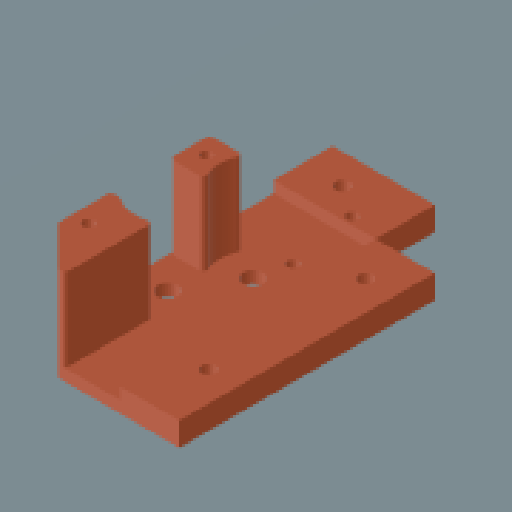
# Autodesk Inventor part: Alpha Idler Assembly
Saved by Autodesk Inventor 2023.2 (Build 272271000, 271)
## iProperties
Created: 2023-02-03
Part Number: Alpha Idler Assembly
Material: ABS Plastic
Document SubType Name: Modeling
Designer: remop
Density: 1.06 g/cm^3
Appearance: Smooth - Light Orange
Author: remop
Autodesk Inventor part; units mm, degrees
ref_plane "YZ Plane" through (0, 0, 0) normal (1, 0, 0) x (0, 1, 0)
ref_plane "XZ Plane" through (0, 0, 0) normal (0, 1, 0) x (-1, 0, 0)
ref_plane "XY Plane" through (0, 0, 0) normal (0, 0, 1) x (1, 0, 0)
sketch "Sketch1" plane through (0, 0, 0) normal (0, 1, 0) x (-1, 0, 0)
  circle A0 centre (25, 36.3) radius 2.5
  circle A1 centre (33, 49.9) radius 2.5
  line L0 (15, 0) -> (15, 15)
  line L1 (15, 15) -> (0, 15)
  line L2 (0, 15) -> (0, 80)
  line L3 (0, 80) -> (41, 80)
  line L4 (41, 80) -> (41, 0)
  line L5 (15, 0) -> (41, 0)
  circle A2 centre (25, 36.3) radius 7.5 construction
  circle A3 centre (33, 49.9) radius 7.5 construction
  point P0 (0, 0)
  dimension "d0" = 5
  dimension "d1" = 15
  dimension "d2" = 25
  dimension "d3" = 21.3
  dimension "d4" = 8
  dimension "d5" = 13.6
  dimension "d12" = 15
  dimension "d46" = 80
  dimension "d47" = 41
  constraints: 12 end point, 6 perpendicular, 4 centre point, 2 coincident, 2 equal radius, 1 horizontal alignment, 1 vertical, 1 vertical alignment
  measures "d0" diameter of A1
  measures "d1" distance of L0.end L1.end
  measures "d2" distance from line of L2 A0.centre
  measures "d3" distance from line of L1 A0.centre
  measures "d4" horizontal distance of A1.centre A0.centre
  measures "d5" vertical distance of A1.centre A0.centre
  measures "d12" diameter of A3
  measures "d46" distance of L3.end L4.end
  measures "d47" distance of L2.end L3.end
extrude "Extrusion1" add sketch "Sketch1" along normal blind 3
sketch "Sketch2" plane through (0, 3, 0) normal (0, 1, 0) x (1, 0, 0)
  line L0 (-41, 0) -> (-41, -80) projected
  line L1 (-41, -80) -> (0, -80) projected
  line L2 (0, -80) -> (0, -15) projected
  line L3 (0, -15) -> (-15, -15) projected
  line L4 (-15, -15) -> (-15, 0) projected
  line L5 (-15, 0) -> (-41, 0) projected
  circle A0 centre (-33, -49.9) radius 2.5 projected
  circle A1 centre (-25, -36.3) radius 2.5 projected
  line L6 (-15, -15) -> (-15, 0) projected
  line L7 (-15, -15) -> (-15, -80)
  line L8 (-15, -15) -> (-41, -15)
  line L9 (-41, 0) -> (-41, -80) projected
  point P0 (0, 0)
  constraints: 4 end point, 3 point on line, 1 perpendicular
extrude "Extrusion2" add sketch "Sketch2" along normal blind 3 contours L5 L4 L8 L0 | L3 L2 L1 L7
sketch "Sketch3" plane through (0, 3, 0) normal (0, 1, 0) x (1, 0, 0)
  circle A0 centre (-25, -36.3) radius 2.5 projected
  circle A1 centre (-33, -49.9) radius 2.5 projected
  line L0 (-15, -80) -> (-15, -15) projected
  line L1 (-15, -15) -> (-41, -15) projected
  line L2 (-41, -15) -> (-41, -80) projected
  line L3 (-41, -80) -> (-15, -80) projected
  circle A2 centre (-25, -36.3) radius 2.5 projected
  circle A3 centre (-25, -36.3) radius 8.5
  circle A4 centre (-33, -49.9) radius 2.5 projected
  circle A5 centre (-33, -49.9) radius 8.5
  line L4 (-31.8739, -31.3) -> (-41, -31.3)
  line L5 (-41, 0) -> (-41, -80) projected
  line L6 (-33, -41.4) -> (-41, -41.4)
  line L7 (-38.3753, -56.4846) -> (-41, -56.4846)
  line L8 (-29, -57.4) -> (-29, -80)
  line L9 (-41, -80) -> (0, -80) projected
  point P0 (0, 0)
  point P1 (-31.727, -41.4959)
  dimension "d15" = 17
  dimension "d16" = 5
  dimension "d19" = 12
  constraints: 8 end point, 4 perpendicular, 4 point on line, 3 point on circle, 2 coincident, 1 centre point, 1 tangent, 4 other
  measures "d16" distance from line of A0.centre L4
  measures "d19" distance between parallel lines of L2 L8
extrude "Extrusion3" add sketch "Sketch3" along normal blind 21 contours L3 L2 L7 A5 L8 | L4 A3 A5 L6 L2
fillet "Fillet1" radius 1 8 edges at (-31.8739, 13.5, 31.3) (-31.727, 13.5, 41.4959) (-41, 13.5, 41.4) (-41, 13.5, 31.3) (-41, 13.5, 56.4846) (-29, 13.5, 57.4) (-29, 13.5, 80) (-38.3753, 13.5, 56.4846)
chamfer "Chamfer1" distance 10 angle 45 1 edges at (-41, 12, 80)
sketch "Sketch4" plane through (0, 24, 0) normal (0, 1, 0) x (1, 0, 0)
  line L0 (-31, -80) -> (-41, -70) projected
  line L1 (-31, -80) -> (-30, -80) projected
  arc A0 (-30, -80) -> (-29, -79) centre (-30, -79) ccw projected
  line L2 (-29, -79) -> (-29, -58.9139) projected
  arc A1 (-29, -58.9139) -> (-30.3158, -57.965) centre (-30, -58.9139) ccw projected
  arc A2 (-38.1184, -56.6862) -> (-30.3158, -57.965) centre (-33, -49.9) ccw projected
  arc A3 (-38.1184, -56.6862) -> (-38.7205, -56.4846) centre (-38.7205, -57.4846) ccw projected
  line L3 (-38.7205, -56.4846) -> (-40, -56.4846) projected
  arc A4 (-40, -56.4846) -> (-41, -57.4846) centre (-40, -57.4846) ccw projected
  line L4 (-41, -57.4846) -> (-41, -70) projected
  arc A5 (-40, -31.3) -> (-41, -32.3) centre (-40, -32.3) ccw projected
  line L5 (-41, -32.3) -> (-41, -40.4) projected
  arc A6 (-41, -40.4) -> (-40, -41.4) centre (-40, -40.4) ccw projected
  line L6 (-40, -41.4) -> (-33.5697, -41.4) projected
  arc A7 (-33.5697, -41.4) -> (-32.6676, -39.9684) centre (-33.5697, -40.4) ccw projected
  arc A8 (-32.7098, -32.7211) -> (-32.6676, -39.9684) centre (-25, -36.3) ccw projected
  arc A9 (-32.7098, -32.7211) -> (-33.6168, -31.3) centre (-33.6168, -32.3) ccw projected
  line L7 (-33.6168, -31.3) -> (-40, -31.3) projected
  point P0 (0, 0)
  point P1 (-37, -36)
  point P2 (-37, -66)
  dimension "d24" = 4
  dimension "d25" = 36
  dimension "d26" = 30
  constraints: 1 vertical alignment
  measures "d24" distance from line of L5 point (-37, -36)
  measures "d25" vertical distance of point (-37, -36) point (0, 0)
  measures "d26" distance of point (-37, -66) point (-37, -36)
hole "Hole1" at (-37, 24, 36) at (-37, 24, 66) direction (0, -1, 0) diameter 2.8 depth 10 tip angle 118
sketch "Sketch5" plane through (0, 0, 0) normal (0, -1, 0) x (1, 0, 0)
  line L0 (-41, 70) -> (-31, 80) projected
  line L1 (-41, 0) -> (-41, 70) projected
  line L2 (-15, 0) -> (-41, 0) projected
  line L3 (-15, 15) -> (-15, 0) projected
  line L4 (0, 15) -> (-15, 15) projected
  line L5 (0, 80) -> (0, 15) projected
  line L6 (-31, 80) -> (0, 80) projected
  circle A0 centre (-33, 49.9) radius 2.5 projected
  circle A1 centre (-25, 36.3) radius 2.5 projected
  point P0 (0, 0)
  point P1 (-31, 7.5)
  point P2 (-7.5, 25)
  point P3 (-7.5, 65)
  dimension "d34" = 7.5
  dimension "d35" = 7.5
  dimension "d36" = 10
  dimension "d37" = 15
  dimension "d38" = 40
  constraints: 1 vertical alignment
  measures "d34" distance from line of L5 point (-7.5, 25)
  measures "d35" distance from line of L2 point (-31, 7.5)
  measures "d36" distance from line of L1 point (-31, 7.5)
  measures "d37" distance from line of L6 point (-7.5, 65)
  measures "d38" distance of point (-7.5, 25) point (-7.5, 65)
hole "Hole2" at (-31, 0, 7.5) at (-7.5, 0, 25) at (-7.5, 0, 65) direction (0, 1, 0) diameter 3.6 end through all counterbore diameter 6.5 counterbore depth 3.4 clearance for "Socket Head Cap Screw ISO 4762" size "M3" standard "ISO"
sketch "Sketch6" plane through (0, 0, 0) normal (0, -1, 0) x (1, 0, 0)
  circle A0 centre (-7.5, 25) radius 3.25 projected
  circle A1 centre (-31, 7.5) radius 3.25 projected
  circle A2 centre (-7.5, 65) radius 3.25 projected
  line L0 (-41, 70) -> (-31, 80) projected
  line L1 (-41, 0) -> (-41, 70) projected
  line L2 (-15, 0) -> (-41, 0) projected
  line L3 (-15, 15) -> (-15, 0) projected
  line L4 (0, 15) -> (-15, 15) projected
  line L5 (0, 80) -> (0, 15) projected
  line L6 (-31, 80) -> (0, 80) projected
  circle A3 centre (-33, 49.9) radius 2.5 projected
  circle A4 centre (-25, 36.3) radius 2.5 projected
  point P0 (0, 0)
  point P1 (-23, 13)
  point P2 (-23, 28)
  dimension "d48" = 15
  dimension "d49" = 8
  dimension "d50" = 13
  constraints: 1 vertical alignment
  measures "d48" distance of point (-23, 13) point (-23, 28)
  measures "d49" distance from line of L3 point (-23, 13)
  measures "d50" distance from line of L2 point (-23, 13)
hole "Hole3" at (-23, 0, 13) at (-23, 0, 28) direction (0, 1, 0) diameter 2.8 end through all
equation "\"d35\" = d34"
body "Solid1"
